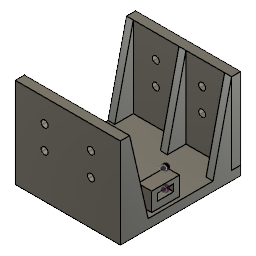
X Carriage (Autodesk Fusion 360 design; units mm, degrees)
Autodesk Fusion 360 part; units mm, degrees
sketch "Skizze1" plane through (0, 0, 0) normal (0, 1, 0) x (1, 0, 0)
  line L0 (0, 0) -> (45.4, 0)
  line L1 (45.4, 0) -> (45.4, -27)
  line L2 (0, 0) -> (0, -27)
  line L3 (0, -27) -> (45.4, -27)
  dimension "d1" = 45.4
  dimension "d2" = 27
  dimension "d3" = 27
  constraint coincident L0.start L2.start
  constraint horizontal L0
  constraint perpendicular L0 L1
  constraint perpendicular L0 L2
  measures "d1" distance of L0.start L0.end
  measures "d2" distance of L0.end L1.end
  measures "d3" distance of L0.start L2.end
extrude "Extrusion1" add sketch "Skizze1" along normal blind 3
sketch "Skizze2" plane through (0, 3, 0) normal (0, 1, 0) x (-1, 0, 0)
  line L0 (0, 0) -> (0, 27)
  line L1 (0, 27) -> (-45.4, 27)
  line L2 (-45.4, 27) -> (-45.4, 0)
  line L3 (-45.4, 0) -> (0, 0)
sketch "Skizze3" plane through (0, 3, 0) normal (0, 1, 0) x (-1, 0, 0)
  circle A0 centre (-32.7, 23.5) radius 1.5
  circle A1 centre (-12.7, 23.5) radius 1.5
  circle A2 centre (-32.7, 3.5) radius 1.5
  circle A3 centre (-12.7, 3.5) radius 1.5
  dimension "d10" = 3
  dimension "d12" = 3
  dimension "d14" = 3
  dimension "d16" = 3
  measures "d10" diameter of A0
  measures "d12" diameter of A1
  measures "d14" diameter of A2
  measures "d16" diameter of A3
extrude "Extrusion2" cut sketch "Skizze3" against normal blind 14
sketch "Skizze4" plane through (0, 3, 0) normal (0, 1, 0) x (-1, 0, 0)
sketch "Skizze5" plane through (0, 3, 0) normal (0, 1, 0) x (-1, 0, 0)
sketch "Skizze6" plane through (0, 0, 0) normal (0, -1, 0) x (1, 0, 0)
  circle A0 centre (32.7, 3.5) radius 1.5
  circle A1 centre (32.7, 23.5) radius 1.5
  circle A2 centre (12.7, 3.5) radius 1.5
  circle A3 centre (12.7, 23.5) radius 1.5
  line L0 (0, 27) -> (0, 0)
  line L1 (0, 0) -> (45.4, 0)
  line L2 (45.4, 0) -> (45.4, 27)
  line L3 (45.4, 27) -> (0, 27)
sketch "Skizze7" plane through (0, 3, 0) normal (0, 1, 0) x (-1, 0, 0)
  line L0 (-45.4, 27) -> (-45.4, 13.5)
  line L1 (-45.4, 13.5) -> (-43.9, 13.5)
  line L2 (-43.9, 13.5) -> (-43.9, 17)
  line L3 (-43.9, 13.5) -> (-43.9, 10)
  line L4 (-43.9, 17) -> (-40.9, 17)
  line L5 (-43.9, 10) -> (-40.9, 10)
  line L6 (-40.9, 17) -> (-40.9, 10)
  line L7 (0, 27) -> (0, 13.5)
  line L8 (0, 13.5) -> (-1.5, 13.5)
  line L9 (-1.5, 13.5) -> (-1.5, 17)
  line L10 (-1.5, 13.5) -> (-1.5, 10)
  line L11 (-1.5, 10) -> (-4.5, 10)
  line L12 (-4.5, 10) -> (-4.5, 17)
  line L13 (-4.5, 17) -> (-1.5, 17)
  dimension "d19" = 13.5
  dimension "d20" = 1.5
  dimension "d21" = 3.5
  dimension "d22" = 3.5
  dimension "d23" = 3
  dimension "d24" = 3
  dimension "d25" = 13.5
  constraint vertical L0
  constraint perpendicular L0 L1
  constraint perpendicular L1 L2
  constraint perpendicular L1 L3
  constraint perpendicular L2 L4
  constraint perpendicular L3 L5
  constraint perpendicular L5 L7
  constraint perpendicular L7 L8
  constraint perpendicular L8 L9
  constraint perpendicular L8 L10
  constraint perpendicular L10 L11
  constraint perpendicular L8 L12
  constraint perpendicular L12 L13
  measures "d19" distance of L0.start L0.end
  measures "d20" distance of L0.end L1.end
  measures "d21" distance of L1.end L2.end
  measures "d22" distance of L1.end L3.end
  measures "d23" distance of L2.end L4.end
  measures "d24" distance of L3.end L5.end
  measures "d25" distance of L7.start L7.end
extrude "Extrusion3" cut sketch "Skizze7" against normal blind 17
sketch "Skizze8" plane through (0, 0, 0) normal (0, -1, 0) x (1, 0, 0)
extrude "Extrusion4" add sketch "Skizze6" along normal blind 1
extrude "Extrusion5" cut sketch "Skizze7" against normal blind 18
sketch "Skizze9" plane through (0, 3, 0) normal (0, 1, 0) x (-1, 0, 0)
  line L0 (-40.9, 10) -> (-43.9, 10)
  line L1 (-43.9, 10) -> (-43.9, 17)
  line L2 (-43.9, 17) -> (-40.9, 17)
  line L3 (-40.9, 17) -> (-40.9, 10)
  line L4 (-4.5, 17) -> (-1.5, 17)
  line L5 (-1.5, 17) -> (-1.5, 10)
  line L6 (-1.5, 10) -> (-4.5, 10)
  line L7 (-4.5, 10) -> (-4.5, 17)
  circle A0 centre (-32.7, 3.5) radius 1.5
  circle A1 centre (-32.7, 23.5) radius 1.5
  circle A2 centre (-12.7, 3.5) radius 1.5
  circle A3 centre (-12.7, 23.5) radius 1.5
  line L8 (0, 0) -> (0, 27)
  line L9 (0, 27) -> (-45.4, 27)
  line L10 (-45.4, 27) -> (-45.4, 0)
  line L11 (-45.4, 0) -> (0, 0)
  circle A4 centre (-12.7, 3.5) radius 2.75
  circle A5 centre (-32.7, 3.5) radius 2.75
  circle A6 centre (-12.7, 23.5) radius 2.75
  circle A7 centre (-32.7, 23.5) radius 2.75
  dimension "d32" = 5.5
  dimension "d33" = 5.5
  dimension "d34" = 5.5
  dimension "d35" = 5.5
  constraint concentric A2 A4
  constraint concentric A0 A5
  constraint concentric A3 A6
  constraint concentric A1 A7
  measures "d32" diameter of A4
  measures "d33" diameter of A5
  measures "d34" diameter of A6
  measures "d35" diameter of A7
extrude "Extrusion6" cut sketch "Skizze9" against normal blind 2 contours A4 | A5 | A6 | A7
extrude "Extrusion7" add 1 faces at (30.2667, 1.6667, 27) along direction (0, 0, 1) blind 5
sketch "Skizze10" plane through (0, 3, 0) normal (0, 1, 0) x (-1, 0, 0)
  circle A0 centre (-12.7, 3.5) radius 2.75
  circle A1 centre (-12.7, 23.5) radius 2.75
  circle A2 centre (-32.7, 3.5) radius 2.75
  circle A3 centre (-32.7, 23.5) radius 2.75
  line L0 (-40.9, 10) -> (-43.9, 10)
  line L1 (-43.9, 10) -> (-43.9, 17)
  line L2 (-43.9, 17) -> (-40.9, 17)
  line L3 (-40.9, 17) -> (-40.9, 10)
  line L4 (-4.5, 17) -> (-1.5, 17)
  line L5 (-1.5, 17) -> (-1.5, 10)
  line L6 (-1.5, 10) -> (-4.5, 10)
  line L7 (-4.5, 10) -> (-4.5, 17)
  line L8 (0, 0) -> (0, 32)
  line L9 (0, 32) -> (-45.4, 32)
  line L10 (-45.4, 32) -> (-45.4, 0)
  line L11 (-45.4, 0) -> (0, 0)
  line L12 (0, 32) -> (0, 28)
  line L13 (-45.4, 28) -> (0, 28)
  line L14 (-45.4, 32) -> (-45.4, 28)
  line L15 (-45.4, 32) -> (0, 32)
  constraint coincident L8.end L9.start
  constraint coincident L8 L12.end
  constraint perpendicular L9 L12
  constraint coincident L10 L13.start
  constraint perpendicular L12 L13
  constraint coincident L9.end L10.start
extrude "Extrusion8" add sketch "Skizze10" along normal blind 35 contours L8 L9 L10 L12 L13 L14 L15
sketch "Skizze11" plane through (0, 0, 32) normal (0, 0, 1) x (1, 0, 0)
  line L0 (45.4, -1) -> (45.4, 38)
  line L1 (45.4, 38) -> (0, 38)
  line L2 (0, 38) -> (0, -1)
  line L3 (0, -1) -> (45.4, -1)
  line L4 (0, -1) -> (0, 3)
  line L5 (0, 38) -> (12.7, 38)
  line L6 (45.4, 38) -> (32.7, 38)
  line L7 (12.7, 38) -> (12.7, 28)
  circle A0 centre (12.7, 28) radius 1.5
  circle A1 centre (12.7, 18) radius 1.5
  circle A2 centre (32.7, 28) radius 1.5
  circle A3 centre (32.7, 18) radius 1.5
  dimension "d42" = 12.7
  dimension "d43" = 12.7
  dimension "d44" = 3
  dimension "d45" = 10
  dimension "d46" = 3
  dimension "d47" = 20
  dimension "d48" = 3
  dimension "d49" = 10
  dimension "d50" = 3
  constraint coincident L2.end L3.start
  constraint coincident L2 L4.end
  constraint coincident L1.end L2.start
  constraint perpendicular L2 L5
  constraint coincident L0.end L1.start
  constraint perpendicular L0 L6
  constraint perpendicular L5 L7
  constraint coincident L7.end A0.centre
  measures "d42" distance of L1.end L5.end
  measures "d43" distance of L0.end L6.end
  measures "d44" diameter of A0
  measures "d45" distance of L7.end A1.centre
  measures "d46" diameter of A1
  measures "d47" distance of L7.end A2.centre
  measures "d48" diameter of A2
  measures "d49" distance of A2.centre A3.centre
  measures "d50" diameter of A3
extrude "Extrusion9" cut sketch "Skizze11" against normal blind 59 contours A0 | A1 | A2 | A3
extrude "Extrusion10" add 1 faces at (30.2667, 0.3333, 0) along direction (0, 0, -1) blind 20
sketch "Skizze12" plane through (0, 3, 0) normal (0, 1, 0) x (-1, 0, 0)
  line L0 (0, 28) -> (-45.4, 28)
  line L1 (-45.4, 28) -> (-45.4, -20)
  line L2 (-45.4, -20) -> (0, -20)
  line L3 (0, -20) -> (0, 28)
  line L4 (-4.5, 17) -> (-1.5, 17)
  line L5 (-1.5, 17) -> (-1.5, 10)
  line L6 (-1.5, 10) -> (-4.5, 10)
  line L7 (-4.5, 10) -> (-4.5, 17)
  line L8 (-40.9, 10) -> (-43.9, 10)
  line L9 (-43.9, 10) -> (-43.9, 17)
  line L10 (-43.9, 17) -> (-40.9, 17)
  line L11 (-40.9, 17) -> (-40.9, 10)
  circle A0 centre (-32.7, 23.5) radius 2.75
  circle A1 centre (-32.7, 3.5) radius 2.75
  circle A2 centre (-12.7, 23.5) radius 2.75
  circle A3 centre (-12.7, 3.5) radius 2.75
  line L12 (0, -20) -> (0, -16)
  line L13 (0, -16) -> (-1, -16)
  line L14 (-1, -16) -> (-45.4, -16)
  line L15 (-45.4, -20) -> (-45.4, -16)
  line L16 (0, -20) -> (-45.4, -20)
  constraint coincident L2.end L3.start
  constraint coincident L3 L12.end
  constraint perpendicular L2 L12
  constraint perpendicular L12 L13
  constraint coincident L1 L14.end
  constraint perpendicular L1 L14
  constraint coincident L1.end L2.start
extrude "Extrusion11" add sketch "Skizze12" along normal blind 35 contours L1 L2 L3 L12 L13 L14 L15 L16
extrude "Extrusion12" cut sketch "Skizze11" against normal blind 77 contours A0 | A1 | A2 | A3
sketch "Skizze13" plane through (0, 0, 28) normal (0, 0, -1) x (-1, 0, 0)
  circle A0 centre (-32.7, 28) radius 1.5
  circle A1 centre (-32.7, 18) radius 1.5
  circle A2 centre (-12.7, 28) radius 1.5
  circle A3 centre (-12.7, 18) radius 1.5
  line L0 (-45.4, 3) -> (0, 3)
  line L1 (0, 3) -> (0, 38)
  line L2 (0, 38) -> (-45.4, 38)
  line L3 (-45.4, 38) -> (-45.4, 3)
  line L4 (-45.4, 38) -> (-42.4, 38)
  line L5 (-45.4, 38) -> (-45.4, 3)
  line L6 (-45.4, 3) -> (-42.4, 3)
  line L7 (-42.4, 38) -> (-42.4, 3)
  dimension "d59" = 3
  dimension "d60" = 3
  constraint coincident L2.end L3.start
  constraint perpendicular L3 L4
  constraint coincident L0.start L3.end
  constraint perpendicular L5 L6
  measures "d59" distance of L2.end L4.end
  measures "d60" distance of L0.start L6.end
extrude "Extrusion13" add sketch "Skizze13" along normal blind 8 contours L0 L2 L3 L4 L5 L6 L7
sketch "Skizze14" plane through (45.4, 0, 0) normal (1, 0, 0) x (0, 0, -1)
  line L0 (20, 3) -> (16, 3)
  line L1 (16, 3) -> (-20, 3)
  line L2 (-20, 3) -> (-20, 38)
  line L3 (-20, 38) -> (-32, 38)
  line L4 (-32, 38) -> (-32, -1)
  line L5 (-32, -1) -> (20, -1)
  line L6 (20, -1) -> (20, 3)
  line L7 (-32, 38) -> (-28, 38)
  line L8 (-28, 38) -> (-20, 3)
  constraint coincident L3.end L4.start
  constraint coincident L3 L7.end
  constraint perpendicular L4 L7
  constraint coincident L1.end L2.start
extrude "Extrusion14" cut sketch "Skizze14" against normal blind 72 contours L2 L3 L8
sketch "Skizze15" plane through (0, 0, 28) normal (0, 0, -1) x (-1, 0, 0)
  line L0 (-42.4, 38) -> (-42.4, 3)
  line L1 (-42.4, 3) -> (0, 3)
  line L2 (0, 3) -> (0, 38)
  line L3 (0, 38) -> (-42.4, 38)
  circle A0 centre (-12.7, 18) radius 1.5
  circle A1 centre (-12.7, 28) radius 1.5
  circle A2 centre (-32.7, 18) radius 1.5
  circle A3 centre (-32.7, 28) radius 1.5
  line L4 (-32.7, 28) -> (-22.7, 28)
  line L5 (-22.7, 28) -> (-22.7, 38)
  line L6 (-22.7, 28) -> (-22.7, 3)
  line L7 (-22.7, 38) -> (-19.7, 38)
  line L8 (-19.7, 38) -> (-19.7, 3)
  line L9 (-19.7, 3) -> (-22.7, 3)
  dimension "d65" = 10
  dimension "d66" = 3
  constraint coincident A3.centre L4.start
  constraint horizontal L4
  constraint coincident L3 L5.end
  constraint perpendicular L3 L5
  constraint coincident L1 L6.end
  constraint perpendicular L1 L6
  constraint perpendicular L5 L7
  constraint coincident L1 L8.end
  constraint perpendicular L1 L8
  measures "d65" distance of A3.centre L4.end
  measures "d66" distance of L5.end L7.end
extrude "Extrusion15" add sketch "Skizze15" along normal blind 8 contours L1 L3 L5 L6 L7 L8 L9
sketch "Skizze16" plane through (0, 0, 32) normal (0, 0, 1) x (1, 0, 0)
sketch "Skizze17" plane through (0, 0, 28) normal (0, 0, -1) x (-1, 0, 0)
  line L0 (-19.7, 38) -> (-19.7, 3)
  line L1 (-19.7, 3) -> (0, 3)
  line L2 (0, 3) -> (0, 38)
  line L3 (0, 38) -> (-19.7, 38)
  circle A0 centre (-12.7, 18) radius 1.5
  circle A1 centre (-12.7, 28) radius 1.5
  line L4 (0, 38) -> (-3, 38)
  line L5 (-3, 38) -> (-3, 3)
  line L6 (-3, 3) -> (0, 3)
  constraint coincident L2.end L3.start
  constraint coincident L3 L4.end
  constraint perpendicular L2 L4
  constraint coincident L1 L5.end
  constraint perpendicular L1 L5
  constraint coincident L1.end L2.start
extrude "Extrusion16" add sketch "Skizze17" along normal blind 8 contours L1 L2 L3 L4 L5 L6
sketch "Skizze18" plane through (0, 0, 0) normal (-1, 0, 0) x (0, 0, 1)
  line L0 (20, 3) -> (-16, 3)
  line L1 (-16, 3) -> (-16, 38)
  line L2 (-16, 38) -> (-20, 38)
  line L3 (-20, 38) -> (-20, -1)
  line L4 (-20, -1) -> (32, -1)
  line L5 (32, -1) -> (32, 38)
  line L6 (32, 38) -> (20, 38)
  line L7 (20, 38) -> (20, 3)
  line L8 (32, 38) -> (28, 38)
  line L9 (28, 38) -> (20, 3)
  constraint coincident L5.end L6.start
  constraint coincident L6 L8.end
  constraint perpendicular L5 L8
  constraint coincident L0.start L7.end
extrude "Extrusion17" cut sketch "Skizze18" against normal blind 67 contours L6 L7 L9
sketch "Skizze19" plane through (0, 0, -16) normal (0, 0, 1) x (1, 0, 0)
  circle A0 centre (32.7, 28) radius 1.5
  circle A1 centre (32.7, 18) radius 1.5
  circle A2 centre (12.7, 28) radius 1.5
  circle A3 centre (12.7, 18) radius 1.5
  line L0 (0, 3) -> (45.4, 3)
  line L1 (45.4, 3) -> (45.4, 38)
  line L2 (45.4, 38) -> (0, 38)
  line L3 (0, 38) -> (0, 3)
  line L4 (0, 38) -> (3, 38)
  line L5 (3, 38) -> (3, 3)
  line L6 (3, 3) -> (0, 3)
  line L7 (0, 38) -> (0, 3)
  line L8 (12.7, 28) -> (22.7, 28)
  line L9 (22.7, 28) -> (22.7, 38)
  line L10 (22.7, 28) -> (22.7, 3)
  line L11 (22.7, 3) -> (25.7, 3)
  line L12 (25.7, 3) -> (25.7, 38)
  line L13 (25.7, 38) -> (22.7, 38)
  line L14 (45.4, 38) -> (42.4, 38)
  line L15 (42.4, 38) -> (42.4, 3)
  line L16 (42.4, 3) -> (45.4, 3)
  dimension "d73" = 10
  dimension "d74" = 3
  dimension "d75" = 3
  constraint coincident L2.end L3.start
  constraint coincident L2 L4.end
  constraint perpendicular L3 L4
  constraint coincident L0 L5.end
  constraint perpendicular L0 L5
  constraint coincident L0.start L3.end
  constraint coincident A2.centre L8.start
  constraint perpendicular L7 L8
  constraint midpoint L2 L9.end
  constraint midpoint L0 L10.end
  constraint perpendicular L10 L11
  constraint coincident L2 L12.end
  constraint perpendicular L2 L12
  constraint coincident L1.end L2.start
  constraint coincident L2 L14.end
  constraint coincident L0 L15.end
  constraint perpendicular L0 L15
  constraint coincident L0.end L1.start
  measures "d73" distance of A2.centre L8.end
  measures "d74" distance of L10.end L11.end
  measures "d75" distance of L1.end L14.end
extrude "Extrusion18" add sketch "Skizze19" along normal blind 8 contours L0 L2 L3 L4 L5 L6 L7 | L0 L2 L9 L10 L11 L12 L13 | L0 L1 L2 L14 L15 L16
sketch "Skizze20" plane through (0, 0, 0) normal (-1, 0, 0) x (0, 0, 1)
  line L0 (28, 38) -> (20, 3)
  line L1 (20, 3) -> (-8, 3)
  line L2 (-8, 3) -> (-8, 38)
  line L3 (-8, 38) -> (-20, 38)
  line L4 (-20, 38) -> (-20, -1)
  line L5 (-20, -1) -> (32, -1)
  line L6 (32, -1) -> (32, 38)
  line L7 (32, 38) -> (28, 38)
  line L8 (-20, 38) -> (-16, 38)
  line L9 (-16, 38) -> (-8, 3)
  constraint coincident L3.end L4.start
  constraint coincident L3 L8.end
  constraint perpendicular L4 L8
  constraint coincident L1.end L2.start
extrude "Extrusion19" cut sketch "Skizze20" against normal blind 64 contours L2 L3 L9
extrude "Extrusion20" add 1 faces at (42.9, 1.6667, 10) along direction (0, 0, 1) blind 7
extrude "Extrusion21" add 1 faces at (2.5, 1.6667, 10) along direction (0, 0, 1) blind 7
sketch "Skizze21" plane through (0, 3, 0) normal (0, 1, 0) x (-1, 0, 0)
  line L0 (-3, -8) -> (0, -8)
  line L1 (0, -8) -> (0, 20)
  line L2 (0, 20) -> (-3, 20)
  line L3 (-3, 20) -> (-3, 28)
  line L4 (-3, 28) -> (-19.7, 28)
  line L5 (-19.7, 28) -> (-19.7, 20)
  line L6 (-19.7, 20) -> (-22.7, 20)
  line L7 (-22.7, 20) -> (-22.7, 28)
  line L8 (-22.7, 28) -> (-42.4, 28)
  line L9 (-42.4, 28) -> (-42.4, 20)
  line L10 (-42.4, 20) -> (-45.4, 20)
  line L11 (-45.4, 20) -> (-45.4, -8)
  line L12 (-45.4, -8) -> (-42.4, -8)
  line L13 (-42.4, -8) -> (-42.4, -16)
  line L14 (-42.4, -16) -> (-25.7, -16)
  line L15 (-25.7, -16) -> (-25.7, -8)
  line L16 (-25.7, -8) -> (-22.7, -8)
  line L17 (-22.7, -8) -> (-22.7, -16)
  line L18 (-22.7, -16) -> (-3, -16)
  line L19 (-3, -16) -> (-3, -8)
  circle A0 centre (-32.7, 23.5) radius 2.75
  circle A1 centre (-32.7, 3.5) radius 2.75
  circle A2 centre (-12.7, 3.5) radius 2.75
  circle A3 centre (-12.7, 23.5) radius 2.75
  line L20 (-1.5, 17) -> (-4.5, 17)
  line L21 (-4.5, 17) -> (-4.5, 10)
  line L22 (-4.5, 10) -> (-1.5, 10)
  line L23 (-1.5, 10) -> (-1.5, 17)
  line L24 (-43.9, 10) -> (-43.9, 17)
  dimension "d84" = 7
  constraint perpendicular L1 L20
  constraint perpendicular L20 L21
  constraint perpendicular L1 L22
  constraint perpendicular L20 L23
  constraint parallel L11 L24
  measures "d84" distance of L24.start L24.end
extrude "Extrusion22" add sketch "Skizze10" sketch "Skizze21" along normal blind 8 contours L0 L1 L2 L3 of sketch 2 contours L20 L21 L22 L23
sketch "Skizze22" plane through (0, 0, 10) normal (0, 0, -1) x (-1, 0, 0)
  line L0 (-43.9, 3) -> (-40.9, 3)
  line L1 (-40.9, 3) -> (-40.9, 11)
  line L2 (-40.9, 11) -> (-43.9, 11)
  line L3 (-43.9, 11) -> (-43.9, 3)
extrude "Extrusion23" add sketch "Skizze22" 1 faces at (3.5, 5.6667, 10) along normal blind 5
sketch "Skizze23" plane through (43.9, 0, 0) normal (1, 0, 0) x (0, 0, -1)
  line L0 (-17, 3) -> (-5, 3)
  line L1 (-5, 3) -> (-5, 11)
  line L2 (-5, 11) -> (-17, 11)
  line L3 (-17, 11) -> (-17, 3)
  line L4 (-17, 11) -> (-17, 9)
  line L5 (-17, 9) -> (-14.5, 9)
  line L6 (-14.5, 9) -> (-14.5, 6)
  line L7 (-14.5, 6) -> (-7.5, 6)
  line L8 (-7.5, 6) -> (-7.5, 9)
  line L9 (-7.5, 9) -> (-14.5, 9)
  dimension "d89" = 2.5
  constraint coincident L2.end L3.start
  constraint coincident L3 L4.end
  constraint perpendicular L2 L4
  constraint perpendicular L1 L5
  constraint perpendicular L2 L6
  constraint perpendicular L6 L7
  constraint perpendicular L7 L8
  constraint perpendicular L6 L9
  measures "d89" distance of L4.end L5.end
extrude "Extrusion24" cut sketch "Skizze23" against normal blind 54 contours L6 L7 L8 L9
extrude "Extrusion25" add 1 faces at (40.9, 4, 9.8333) along direction (-1, 0, 0) blind 3
extrude "Extrusion26" add 1 faces at (4.5, 4, 12.1667) along direction (1, 0, 0) blind 3
sketch "Skizze24" plane through (37.9, 0, 0) normal (-1, 0, 0) x (0, 0, 1)
  line L0 (14.5, 9) -> (14.5, 6)
  line L1 (14.5, 6) -> (7.5, 6)
  line L2 (7.5, 6) -> (7.5, 9)
  line L3 (7.5, 9) -> (14.5, 9)
  line L4 (5, 3) -> (17, 3)
  line L5 (17, 3) -> (17, 11)
  line L6 (17, 11) -> (5, 11)
  line L7 (5, 11) -> (6, 11)
  line L8 (5, 3) -> (6, 3)
  constraint coincident L6.end L7.start
  constraint coincident L6 L7.end
  constraint coincident L4.start L8.start
  constraint coincident L4 L8.end
sketch "Skizze25" plane through (37.9, 0, 0) normal (-1, 0, 0) x (0, 0, 1)
  line L0 (14.5, 9) -> (14.5, 6)
  line L1 (14.5, 6) -> (7.5, 6)
  line L2 (7.5, 6) -> (7.5, 9)
  line L3 (7.5, 9) -> (14.5, 9)
  line L4 (5, 3) -> (17, 3)
  line L5 (17, 3) -> (17, 11)
  line L6 (17, 11) -> (5, 11)
  line L7 (5, 11) -> (5, 3)
  line L8 (5, 11) -> (7, 11)
  line L9 (7, 11) -> (7, 3)
  line L10 (5, 3) -> (7, 3)
  line L11 (5, 3) -> (5, 11)
  line L12 (17, 11) -> (15, 11)
  line L13 (15, 11) -> (15, 3)
  line L14 (15, 3) -> (17, 3)
  line L15 (17, 3) -> (17, 11)
  constraint coincident L6.end L7.start
  constraint coincident L6 L8.end
  constraint perpendicular L2 L8
  constraint perpendicular L6 L9
  constraint coincident L4.start L7.end
  constraint coincident L5.end L6.start
  constraint coincident L6 L12.end
  constraint perpendicular L5 L12
  constraint perpendicular L6 L13
  constraint coincident L4.end L5.start
extrude "Extrusion27" add sketch "Skizze25" along normal blind 2 contours L4 L6 L7 L8 L9 L10 L11 | L4 L5 L6 L12 L13 L14 L15
sketch "Skizze26" plane through (0, 0, 5) normal (0, 0, -1) x (-1, 0, 0)
  line L0 (-43.9, 11) -> (-43.9, 3)
  line L1 (-43.9, 3) -> (-35.9, 3)
  line L2 (-35.9, 3) -> (-35.9, 11)
  line L3 (-35.9, 11) -> (-43.9, 11)
  line L4 (-35.9, 3) -> (-38, 11)
  constraint coincident L1.end L2.start
  constraint coincident L3 L4.end
extrude "Extrusion28" cut sketch "Skizze26" against normal blind 16 contours L2 L3 L4
sketch "Skizze27" plane through (7.5, 0, 0) normal (1, 0, 0) x (0, 0, -1)
  line L0 (-14.5, 6) -> (-14.5, 9)
  line L1 (-14.5, 9) -> (-7.5, 9)
  line L2 (-7.5, 9) -> (-7.5, 6)
  line L3 (-7.5, 6) -> (-14.5, 6)
  line L4 (-17, 3) -> (-5, 3)
  line L5 (-5, 3) -> (-5, 11)
  line L6 (-5, 11) -> (-17, 11)
  line L7 (-17, 11) -> (-17, 3)
  line L8 (-17, 11) -> (-15, 11)
  line L9 (-15, 11) -> (-15, 3)
  line L10 (-15, 3) -> (-17, 3)
  line L11 (-5, 11) -> (-7, 11)
  line L12 (-7, 11) -> (-7, 3)
  line L13 (-7, 3) -> (-5, 3)
  constraint coincident L6.end L7.start
  constraint coincident L6 L8.end
  constraint perpendicular L7 L8
  constraint coincident L4 L9.end
  constraint perpendicular L4 L9
  constraint coincident L4.start L7.end
  constraint coincident L5.end L6.start
  constraint coincident L6 L11.end
  constraint perpendicular L5 L11
  constraint coincident L4 L12.end
  constraint perpendicular L4 L12
  constraint coincident L4.end L5.start
extrude "Extrusion29" add sketch "Skizze27" along normal blind 2 contours L4 L6 L7 L8 L9 L10 | L4 L5 L6 L11 L12 L13
sketch "Skizze28" plane through (0, 0, 0) normal (1, 0, 0) x (0, 0, -1)
sketch "Skizze29" plane through (0, 0, 5) normal (0, 0, -1) x (-1, 0, 0)
  line L0 (-9.5, 3) -> (-1.5, 3)
  line L1 (-1.5, 3) -> (-1.5, 11)
  line L2 (-1.5, 11) -> (-9.5, 11)
  line L3 (-9.5, 11) -> (-9.5, 3)
  line L4 (-9.5, 3) -> (-7, 11)
  constraint coincident L0.start L3.end
  constraint coincident L2 L4.end
extrude "Extrusion30" cut sketch "Skizze29" against normal blind 13 contours L2 L3 L4
